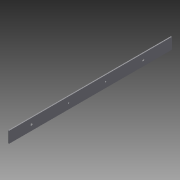
# Autodesk Inventor part: side
Saved by Autodesk Inventor 2015 (Build 190159000, 159)
## iProperties
Created: 2014-11-02
Part Number: side
Material: Generic
Document SubType Name: Modeling
Designer: jesse
Density: 1 g/cm^3
Appearance: Default
Author: jesse
Autodesk Inventor part; units mm, degrees
ref_plane "YZ Plane" through (0, 0, 0) normal (1, 0, 0) x (0, 1, 0)
ref_plane "XZ Plane" through (0, 0, 0) normal (0, 1, 0) x (-1, 0, 0)
ref_plane "XY Plane" through (0, 0, 0) normal (0, 0, 1) x (1, 0, 0)
sketch "Sketch1" plane through (0, 0, 0) normal (1, 0, 0) x (0, 1, 0)
  line L0 (0, 0) -> (38.1, 0)
  line L1 (38.1, 0) -> (38.1, -550.8625)
  line L2 (38.1, -550.8625) -> (0, -550.8625)
  line L3 (0, -550.8625) -> (0, 0)
  line L4 (19.05, 0) -> (19.05, -550.8625) construction
  line L5 (38.1, -76.2) -> (0, -76.2) construction
  line L6 (38.1, -201.6125) -> (0, -201.6125) construction
  line L7 (38.1, -327.025) -> (0, -327.025) construction
  line L8 (38.1, -454.025) -> (0, -454.025) construction
  circle A0 centre (19.05, -201.6125) radius 2.413
  circle A1 centre (19.05, -327.025) radius 2.413
  circle A2 centre (19.05, -76.2) radius 3.9688
  circle A3 centre (19.05, -454.025) radius 3.9687
  dimension "d0" = 38.1
  dimension "d1" = 550.8625
  dimension "d2" = 76.2
  dimension "d3" = 201.6125
  dimension "d4" = 327.025
  dimension "d5" = 454.025
  dimension "d6" = 4.826
  dimension "d7" = 4.826
  dimension "d8" = 7.9375
  dimension "d9" = 7.9375
  constraints: 18 end point, 8 point on line, 6 midpoint, 5 perpendicular, 4 centre point, 2 parallel, 1 horizontal
  measures "d0" distance of L1.end L2.end
  measures "d1" distance of L0.end L1.end
  measures "d2" distance from line of L0 L5.end
  measures "d3" distance between parallel lines of L0 L6
  measures "d4" distance between parallel lines of L7 L0
  measures "d5" distance between parallel lines of L8 L0
  measures "d6" diameter of A0
  measures "d7" diameter of A1
  measures "d8" diameter of A2
  measures "d9" diameter of A3
extrude "Extrusion1" add sketch "Sketch1" along normal blind 3.302
body "Solid1"
